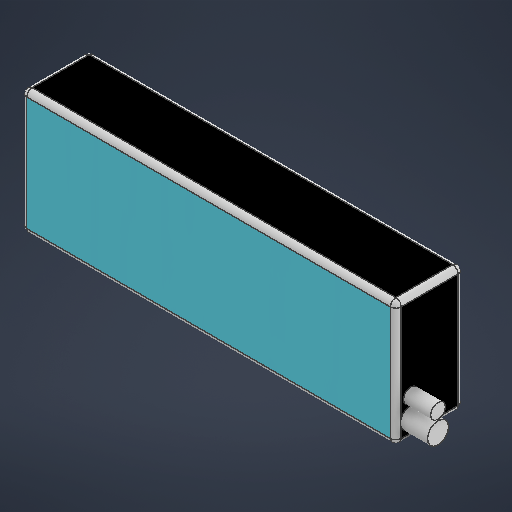
# Autodesk Inventor part: battery1
Saved by Autodesk Inventor 2026.1 (Build 301233000, 233)
## iProperties
Created: 2025-11-06
Part Number: battery1
Material: Generic
Document SubType Name: Modeling
Designer: emanuel
Density: 1 g/cm^3
Appearance: Default
Author: emanuel
Autodesk Inventor part; units mm, degrees
ref_plane "YZ Plane" through (0, 0, 0) normal (1, 0, 0) x (0, 1, 0)
ref_plane "XZ Plane" through (0, 0, 0) normal (0, 1, 0) x (-1, 0, 0)
ref_plane "XY Plane" through (0, 0, 0) normal (0, 0, 1) x (1, 0, 0)
sketch "Sketch1" plane through (0, 0, 0) normal (1, 0, 0) x (0, 1, 0)
  line L0 (0, 0) -> (46, 0)
  line L1 (46, 0) -> (46, -25)
  line L2 (46, -25) -> (0, -25)
  line L3 (0, -25) -> (0, 0)
  dimension "d0" = 46
  dimension "d1" = 25
  constraints: 8 end point, 2 parallel, 1 horizontal, 1 perpendicular
  measures "d0" distance of L1.end L2.end
  measures "d1" distance of L0.end L1.end
extrude "Extrusion1" add sketch "Sketch1" along normal blind 138
sketch "Sketch2" plane through (138, 0, 0) normal (1, 0, 0) x (0, 0, -1)
  circle A0 centre (5.5887, 7.0177) radius 3.879
  circle A1 centre (5.5887, 14.0045) radius 2.7237
  point P0 (0, 0)
  constraints: 2 centre point
extrude "Extrusion2" add sketch "Sketch2" along normal blind 10
fillet "Fillet1" radius 2 12 edges at (69, 46, 0) (138, 46, -12.5) (69, 46, -25) (138, 23, 0) (138, 23, -25) (69, 0, 0) (0, 23, 0) (0, 23, -25) (0, 46, -12.5) (138, 0, -12.5) (69, 0, -25) (0, 0, -12.5)
body "Solid1"
